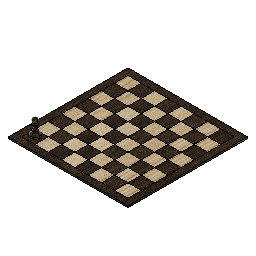
Day8 - Chess board (Autodesk Fusion 360 design; units mm, degrees)
Autodesk Fusion 360 part; units mm, degrees
note: some values were not read from the file. Chosen so that the rebuilt part matches the saved one: which bodies a step acts on.
sketch "Sketch1" plane through (0, 0, 0) normal (0, 0, 1) x (1, 0, 0) in component "Board"
  line L0 (0, 0) -> (40, 0)
  line L1 (40, 0) -> (40, 40)
  line L2 (40, 40) -> (0, 40)
  line L3 (0, 40) -> (0, 0)
  line L4 (40, 40) -> (80, 40)
  line L5 (80, 40) -> (80, 0)
  line L6 (80, 0) -> (40, 0)
  line L7 (40, 0) -> (40, 40)
  line L8 (0, 40) -> (40, 40)
  line L9 (40, 40) -> (40, 80)
  line L10 (40, 80) -> (0, 80)
  line L11 (0, 80) -> (0, 40)
  line L12 (40, 80) -> (80, 80)
  line L13 (80, 80) -> (80, 40)
  line L14 (80, 40) -> (40, 40)
  line L15 (40, 40) -> (40, 80)
  dimension "d1" = 40
  dimension "d2" = 40
  dimension "d3" = 40
  dimension "d4" = 40
extrude "Extrude1" add sketch "Sketch1" along normal blind 5 contours L0 L1 L2 L3 L7 L8 makes body 1 in component "Board"
extrude "Extrude2" add sketch "Sketch1" along normal blind 5 separate body contours L2 L8 L9 L10 L11 L15 makes body 2 in component "Board"
extrude "Extrude3" add sketch "Sketch1" along normal blind 5 separate body contours L1 L4 L5 L6 L7 L14 makes body 3 in component "Board"
extrude "Extrude4" add sketch "Sketch1" along normal blind 5 separate body contours L4 L9 L12 L13 L14 L15 makes body 4 in component "Board"
pattern_linear "R-Pattern1" count 4 spacing 80 along (1, 0, 0) count 4 spacing 80 along (0, 1, 0) of bodies 2 4 1 3 makes body 5 at (93.3333, 66.6667, 0) makes body 6 at (173.3333, 66.6667, 0) makes body 7 at (253.3333, 66.6667, 0) makes body 8 at (13.3333, 146.6667, 0) makes body 9 at (93.3333, 146.6667, 0) makes body 10 at (173.3333, 146.6667, 0) makes body 11 at (253.3333, 146.6667, 0) makes body 12 at (13.3333, 226.6667, 0) makes body 13 at (93.3333, 226.6667, 0) makes body 14 at (173.3333, 226.6667, 0) makes body 15 at (253.3333, 226.6667, 0) makes body 16 at (13.3333, 306.6667, 0) makes body 17 at (93.3333, 306.6667, 0) makes body 18 at (173.3333, 306.6667, 0) makes body 19 at (253.3333, 306.6667, 0) makes body 20 at (133.3333, 26.6667, 0) makes body 21 at (213.3333, 26.6667, 0) makes body 22 at (293.3333, 26.6667, 0) makes body 23 at (53.3333, 106.6667, 0) makes body 24 at (133.3333, 106.6667, 0) makes body 25 at (213.3333, 106.6667, 0) makes body 26 at (293.3333, 106.6667, 0) makes body 27 at (53.3333, 186.6667, 0) makes body 28 at (133.3333, 186.6667, 0) makes body 29 at (213.3333, 186.6667, 0) makes body 30 at (293.3333, 186.6667, 0) makes body 31 at (53.3333, 266.6667, 0) makes body 32 at (133.3333, 266.6667, 0) makes body 33 at (213.3333, 266.6667, 0) makes body 34 at (293.3333, 266.6667, 0) makes body 35 at (93.3333, 26.6667, 0) makes body 36 at (173.3333, 26.6667, 0) makes body 37 at (253.3333, 26.6667, 0) makes body 38 at (13.3333, 106.6667, 0) makes body 39 at (93.3333, 106.6667, 0) makes body 40 at (173.3333, 106.6667, 0) makes body 41 at (253.3333, 106.6667, 0) makes body 42 at (13.3333, 186.6667, 0) makes body 43 at (93.3333, 186.6667, 0) makes body 44 at (173.3333, 186.6667, 0) makes body 45 at (253.3333, 186.6667, 0) makes body 46 at (13.3333, 266.6667, 0) makes body 47 at (93.3333, 266.6667, 0) makes body 48 at (173.3333, 266.6667, 0) makes body 49 at (253.3333, 266.6667, 0) makes body 50 at (133.3333, 66.6667, 0) makes body 51 at (213.3333, 66.6667, 0) makes body 52 at (293.3333, 66.6667, 0) makes body 53 at (53.3333, 146.6667, 0) makes body 54 at (133.3333, 146.6667, 0) makes body 55 at (213.3333, 146.6667, 0) makes body 56 at (293.3333, 146.6667, 0) makes body 57 at (53.3333, 226.6667, 0) makes body 58 at (133.3333, 226.6667, 0) makes body 59 at (213.3333, 226.6667, 0) makes body 60 at (293.3333, 226.6667, 0) makes body 61 at (53.3333, 306.6667, 0) makes body 62 at (133.3333, 306.6667, 0) makes body 63 at (213.3333, 306.6667, 0) makes body 64 at (293.3333, 306.6667, 0) in component "Board"
sketch "Sketch2" plane through (0, 0, 0) normal (0, 0, 1) x (1, 0, 0) in component "Board"
  line L0 (0, 320) -> (320, 320)
  line L1 (320, 320) -> (320, 0)
  line L2 (320, 0) -> (0, 0)
  line L3 (0, 0) -> (0, 320)
  line L4 (340, -20) -> (-20, -20)
  line L5 (-20, -20) -> (-20, 340)
  line L6 (-20, 340) -> (340, 340)
  line L7 (340, 340) -> (340, -20)
  point P0 (0, 20)
  point P1 (20, 0)
  dimension "d17" = 20
  measures "d17" distance of L2
extrude "Extrude5" add sketch "Sketch2" along normal blind 5 separate body makes body 65 in component "Board"
sketch "Sketch1 (2)" plane through (0, 0, 0) normal (0, 1, 0) x (1, 0, 0) in component "Pawn"
  line L0 (0.076, -5.2053) -> (9.6827, -5.2053)
  line L1 (9.6827, -5.2053) -> (13.8853, -8.9536)
  line L2 (13.8853, -8.9536) -> (11.3279, -10.8782)
  spline S0 degree 5 poles (11.3279, -10.8782) (11.6043, -11.1279) (12.0933, -11.6207) (12.6352, -12.3408) (12.9884, -13.2609) (12.8992, -14.3379) (12.3987, -15.3358) (11.6279, -16.2541) (10.7364, -17.1018) (9.8726, -17.9036) (9.1693, -18.701) (8.7226, -19.533) (8.5589, -20.4124) (8.6272, -21.3169) (8.7246, -22.1429) (8.5752, -22.7451) (8.1879, -23.0128) (7.7295, -23.0848) (7.3506, -23.0765) (7.1428, -23.0582) knots 0 0 0 0 0 0 0.066667 0.133333 0.2 0.266667 0.333333 0.4 0.466667 0.533333 0.6 0.666667 0.733333 0.8 0.866667 0.933333 1 1 1 1 1 1
  line L3 (8.5378, -19.9998) -> (8.7524, -22.8973)
  line L4 (9.6646, -9.3759) -> (12.9913, -12.3806)
  spline S1 degree 5 poles (7.1428, -23.0582) (6.8804, -23.3482) (6.3708, -23.9619) (5.6521, -24.9831) (4.7915, -26.5605) (3.9583, -29.0674) (3.608, -31.771) (3.6124, -34.3886) (3.7531, -36.4378) (3.8579, -37.5385) knots 0 0 0 0 0 0 0.2 0.4 0.6 0.8 1 1 1 1 1 1
  line L5 (3.5971, -34.8004) -> (4.1187, -40.2765)
  line L6 (3.8579, -37.5385) -> (7.4652, -37.5385)
  line L7 (7.4652, -37.5385) -> (7.4652, -39.3672)
  line L8 (7.4652, -39.3672) -> (2.9926, -42.1028)
  line L9 (0.076, -5.2053) -> (0.076, -56.1079)
  spline S2 degree 5 poles (0.076, -56.1079) (0.9927, -56.1079) (2.7041, -55.9399) (4.9047, -55.1847) (7.1154, -53.3135) (8.4275, -50.0417) (7.8108, -47.0044) (6.0038, -44.5964) (4.1111, -42.9422) (2.9926, -42.1028) knots 0 0 0 0 0 0 0.2 0.4 0.6 0.8 1 1 1 1 1 1
  line L10 (5.2075, -43.7649) -> (0.7778, -40.4407)
  line L11 (-1.5962, -56.1079) -> (1.7481, -56.1079)
revolve "Revolve1" add sketch "Sketch1 (2)" angle 360 about axis through (0.076, 0, 5.2053) along (0, 0, 1) separate body makes body 66 in component "Pawn"
component "Board" placed x (1, 0, 0) y (0, 1, 0) z (0, 0, 1) at (0, 0, 0)
component "Pawn" placed x (1, 0, 0) y (0, 1, 0) z (0, 0, 1) at (19.924, 20, -0.2053)
